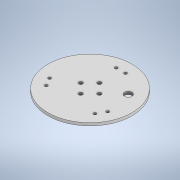
# Autodesk Inventor part: base-3dp
Saved by Autodesk Inventor 2021 (Build 250183000, 183)
## iProperties
Created: 2021-03-27
Part Number: base-3dp
Material: Generic
Document SubType Name: Modeling
Designer: ASUS
Density: 1 g/cm^3
Appearance: Default
Author: ASUS
Autodesk Inventor part; units mm, degrees
ref_plane "YZ Plane" through (0, 0, 0) normal (1, 0, 0) x (0, 1, 0)
ref_plane "XZ Plane" through (0, 0, 0) normal (0, 1, 0) x (-1, 0, 0)
ref_plane "XY Plane" through (0, 0, 0) normal (0, 0, 1) x (1, 0, 0)
sketch "Sketch1" plane through (0, 0, 0) normal (0, 1, 0) x (-1, 0, 0)
  circle A0 centre (0, 0) radius 45
  circle A1 centre (10, 0) radius 2.1
  circle A2 centre (0, 10) radius 2.1
  circle A3 centre (-10, 0) radius 2.1
  circle A4 centre (0, -10) radius 2.1
  dimension "d0" = 90
  dimension "d1" = 10
  dimension "d2" = 4.2
  dimension "d5" = 360
  constraints: 5 centre point, 1 coincident, 1 horizontal alignment, 9 other
  measures "d0" diameter of A0
  measures "d1" distance of point (0, 0) A1.centre
  measures "d2" diameter of A1
extrude "Extrusion1" add sketch "Sketch1" along normal blind 3
sketch "Sketch2" plane through (0, 3, 0) normal (0, 1, 0) x (1, 0, 0)
  circle A0 centre (-5, 33) radius 1.6
  circle A1 centre (5, 33) radius 1.6
  point P0 (0, 0)
  dimension "d9" = 5
  dimension "d10" = 10
  dimension "d11" = 3.2
  dimension "d12" = 33
  constraints: 2 centre point, 1 equal radius, 1 horizontal alignment
  measures "d9" horizontal distance of point (0, 0) A0.centre
  measures "d10" distance of A0.centre A1.centre
  measures "d11" diameter of A1
  measures "d12" vertical distance of point (0, 0) A0.centre
extrude "Extrusion2" cut sketch "Sketch2" against normal up to surface (3 mm away)
pattern_circular "Circular Pattern1" count 3 over 360 about axis through (0, 0, 0) along (0, 1, 0) of "Extrusion2"
sketch "Sketch3" plane through (0, 3, 0) normal (0, 1, 0) x (1, 0, 0)
  circle A0 centre (25.9808, 15) radius 4
  line L0 (25.9808, 15) -> (0, 0) construction
  line L1 (0, 0) -> (24.7895, 0) construction
  dimension "d18" = 8
  dimension "d19" = 30
  dimension "d20" = 30
  constraints: 4 end point, 1 centre point, 1 horizontal
  measures "d18" diameter of A0
  measures "d19" distance of L0.end L0.start
  measures "d20" angle of L0 L1
extrude "Extrusion3" cut sketch "Sketch3" against normal up to surface (3 mm away)
equation "\"d10\" = 2 * d9"
body "Solid1"
